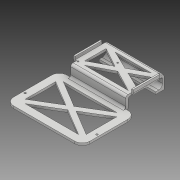
# Autodesk Inventor part: soporte_ubiquiti_usb
Saved by Autodesk Inventor 2018 (Build 220112000, 112)
## iProperties
Created: 2019-01-16
Part Number: soporte_ubiquiti_usb
Material: Genérico
Document SubType Name: Modeling
Designer: becar
Density: 1 g/cm^3
Appearance: Valor por defecto
Author: becar
Autodesk Inventor part; units mm, degrees
ref_plane "YZ Plane" through (0, 0, 0) normal (1, 0, 0) x (0, 1, 0)
ref_plane "XZ Plane" through (0, 0, 0) normal (0, 1, 0) x (-1, 0, 0)
ref_plane "XY Plane" through (0, 0, 0) normal (0, 0, 1) x (1, 0, 0)
sketch "Boceto1" plane through (0, 0, 0) normal (0, 0, 1) x (1, 0, 0)
  line L0 (0, 0) -> (100, 0)
  line L1 (100, 0) -> (100, 70)
  line L2 (100, 70) -> (0, 70)
  line L3 (0, 70) -> (0, 0)
  line L4 (0, 0) -> (0, 22)
  line L5 (100, 0) -> (100, 22)
  circle A0 centre (3, 22) radius 1.25
  circle A1 centre (97, 22) radius 1.25
  line L6 (0, 70) -> (10, 70)
  line L7 (100, 0) -> (90, 0)
  line L8 (90, 0) -> (90, 10)
  line L9 (10, 70) -> (10, 60)
  line L10 (100, 70) -> (90, 70)
  line L11 (90, 70) -> (90, 60)
  line L12 (0, 0) -> (10, 0)
  line L13 (15, 60) -> (85, 60)
  line L14 (15, 10) -> (85, 10)
  line L15 (10, 15) -> (10, 55)
  line L16 (90, 15) -> (90, 55)
  line L17 (10, 55) -> (43.3333, 35)
  line L18 (10, 15) -> (43.3333, 35)
  line L19 (50, 39) -> (15, 60)
  line L20 (50, 39) -> (85, 60)
  line L21 (90, 55) -> (56.6667, 35)
  line L22 (56.6667, 35) -> (90, 15)
  line L23 (85, 10) -> (50, 31)
  line L24 (50, 31) -> (15, 10)
  dimension "d0" = 100
  dimension "d1" = 70
  dimension "d2" = 22
  dimension "d4" = 22
  dimension "d6" = 2.5
  dimension "d7" = 2.5
  dimension "d8" = 10
  dimension "d9" = 10
  dimension "d10" = 10
  dimension "d11" = 10
  dimension "d12" = 5
  dimension "d13" = 5
  dimension "d14" = 5
  dimension "d15" = 5
  dimension "d16" = 10
  constraints: 50 end point, 6 perpendicular, 6 point on line, 2 centre point, 1 collinear, 1 horizontal, 1 vertical
  measures "d0" distance of L0.start L0.end
  measures "d1" distance of L0.end L1.end
  measures "d2" distance of L0.start L4.end
  measures "d4" distance of L0.end L5.end
  measures "d6" diameter of A0
  measures "d7" diameter of A1
  measures "d8" distance of L2.end L6.end
  measures "d9" distance of L0.end L7.end
  measures "d10" distance of L7.end L8.end
  measures "d11" distance of L6.end L9.end
  measures "d12" distance of L9.end L15.end
  measures "d13" distance of L8.end L14.end
  measures "d14" distance of L9.end L13.start
  measures "d15" distance of L8.end L16.start
  measures "d16" distance of L1.end L10.end
extrude "Extrusión1" add sketch "Boceto1" along normal blind 3
sketch "Boceto2" plane through (100, 0, 0) normal (1, 0, 0) x (0, 0, -1)
  line L0 (-3, 70) -> (-3, 0) projected
  line L1 (-3, 70) -> (-18, 70)
  line L2 (-18, 70) -> (-18, 120)
  line L3 (-18, 120) -> (0, 120)
  line L4 (0, 120) -> (0, 117)
  line L5 (0, 117) -> (0, 109)
  line L6 (0, 109) -> (-3, 109)
  line L7 (-3, 109) -> (-3, 117)
  line L8 (-3, 117) -> (-15, 117)
  line L9 (-15, 117) -> (-15, 73)
  line L10 (-15, 73) -> (0, 73)
  line L11 (0, 73) -> (0, 70)
  line L12 (0, 70) -> (-3, 70) projected
  line L13 (0, 70) -> (-3, 70)
  point P0 (0, 0)
  dimension "d25" = 15
  dimension "d26" = 50
  dimension "d27" = 3
  dimension "d28" = 8
  dimension "d29" = 3
  dimension "d30" = 12
  dimension "d31" = 44
  constraints: 24 end point, 6 perpendicular, 3 point on line, 2 vertical, 1 collinear, 1 horizontal
  measures "d25" distance of L0.start L1.end
  measures "d26" distance of L1.end L2.end
  measures "d27" distance of L3.end L4.end
  measures "d28" distance of L4.end L5.end
  measures "d29" distance of L5.end L6.end
  measures "d30" distance of L7.end L8.end
  measures "d31" distance of L8.end L9.end
extrude "Extrusión2" add sketch "Boceto2" against normal up to surface (100 mm away)
sketch "Boceto3" plane through (100, 70, 18) normal (0, 0, 1) x (1, 0, 0)
  line L0 (0, 50) -> (-100, 50) projected
  line L1 (-50, 50) -> (-87, 50)
  line L2 (-87, 50) -> (-87, -0.2579)
  line L3 (-87, -0.2579) -> (-100, -0.2579)
  line L4 (-100, -0.2579) -> (-100, 50)
  line L5 (-100, 50) -> (-87, 50)
  line L6 (-50, 50) -> (-13, 50)
  line L7 (-13, 50) -> (-13, -0.2579)
  line L8 (-13, -0.2579) -> (0, -0.2579)
  line L9 (0, -70) -> (0, 3) projected
  line L10 (0, -0.2579) -> (0, 50)
  line L11 (-13, 50) -> (0, 50)
  point P0 (-100, -70)
  dimension "d34" = 37
  dimension "d35" = 37
  constraints: 20 end point, 7 perpendicular, 3 point on line, 1 horizontal, 1 midpoint
  measures "d34" distance of L1.start L1.end
  measures "d35" distance of L1.start L6.end
extrude "Extrusión3" cut sketch "Boceto3" against normal up to surface (18 mm away)
sketch "Boceto4" plane through (13, 120, 18) normal (0, 0, 1) x (1, 0, 0)
  line L0 (0, 0) -> (0, -50) projected
  line L1 (0, -25) -> (0, -7.5)
  line L2 (0, -7.5) -> (-2, -7.5)
  line L3 (-2, -7.5) -> (-2, -42.5)
  line L4 (-2, -42.5) -> (0, -42.5)
  line L5 (0, -42.5) -> (0, -25)
  line L6 (74, -50) -> (74, 0) projected
  line L7 (74, -25) -> (74, -7.5)
  line L8 (74, -7.5) -> (76, -7.5)
  line L9 (76, -7.5) -> (76, -42.5)
  line L10 (76, -42.5) -> (74, -42.5)
  line L11 (74, -42.5) -> (74, -25)
  point P0 (-13, -120)
  dimension "d38" = 17.5
  dimension "d39" = 2
  dimension "d40" = 35
  dimension "d41" = 2
  constraints: 20 end point, 6 perpendicular, 4 point on line, 2 collinear, 2 midpoint
  measures "d38" distance of L1.start L1.end
  measures "d39" distance of L1.end L2.end
  measures "d40" distance of L2.end L3.end
  measures "d41" distance of L7.end L8.end
extrude "Extrusión4" add sketch "Boceto4" along normal blind 4
sketch "Boceto5" plane through (87, 77.5, 18) normal (0, -1, 0) x (1, 0, 0)
  line L0 (-76, 0) -> (-76, -3)
  line L1 (0, -3) -> (-74, -3) projected
  line L2 (-76, -3) -> (-74, -3)
  line L3 (0, 0) -> (-74, 0) projected
  line L4 (-74, -3) -> (-74, 0)
  line L5 (0, 0) -> (2, 0) projected
  line L6 (2, 0) -> (2, -3)
  line L7 (0, -3) -> (0, -18) projected
  line L8 (2, -3) -> (0, -3)
  line L9 (0, -3) -> (0, 0)
  line L10 (0, 0) -> (2, 0)
  line L11 (-76, 0) -> (-76, 4) projected
  line L12 (-76, 0) -> (-74, 0) projected
  line L13 (-76, 0) -> (-74, 0)
  point P0 (-87, -18)
  dimension "d44" = 3
  constraints: 16 end point, 4 perpendicular, 2 vertical, 1 collinear
  measures "d44" distance of L0.start L0.end
extrude "Extrusión5" add sketch "Boceto5" against normal up to surface (35 mm away) contours L12 L4 L2 L0 | L5 L6 L8 L9
sketch "Boceto6" plane through (13, 120, 18) normal (0, 0, 1) x (1, 0, 0)
  line L0 (74, 0) -> (0, 0) projected
  line L1 (37, 0) -> (1.25, 0)
  line L2 (37, 0) -> (72.75, 0)
  line L3 (72.75, 0) -> (72.75, -47)
  line L4 (74, -47) -> (0, -47) projected
  line L5 (72.75, -23.5) -> (72.75, -2)
  line L6 (72.75, -23.5) -> (72.75, -45)
  line L7 (72.75, -45) -> (1.25, -45)
  line L8 (1.25, -45) -> (1.25, -2)
  line L9 (1.25, -2) -> (72.75, -2)
  line L10 (1.25, -2) -> (1.25, -18)
  line L11 (1.25, -18) -> (31.25, -18)
  circle A0 centre (31.25, -18) radius 1
  line L12 (1.25, -45) -> (3.75, -45)
  line L13 (3.75, -45) -> (3.75, -42.5)
  circle A1 centre (3.75, -42.5) radius 1
  line L14 (72.75, -2) -> (71.25, -2)
  line L15 (71.25, -2) -> (71.25, -3.5)
  circle A2 centre (71.25, -3.5) radius 1
  point P0 (-13, -120)
  dimension "d47" = 35.75
  dimension "d48" = 35.75
  dimension "d49" = 21.5
  dimension "d50" = 21.5
  dimension "d52" = 16
  dimension "d53" = 30
  dimension "d54" = 2
  dimension "d55" = 2.5
  dimension "d56" = 2.5
  dimension "d57" = 2
  dimension "d58" = 1.5
  dimension "d59" = 1.5
  dimension "d60" = 2
  constraints: 28 end point, 8 point on line, 6 perpendicular, 3 centre point, 3 coincident, 2 midpoint
  measures "d47" distance of L1.start L1.end
  measures "d48" distance of L1.start L2.end
  measures "d49" distance of L5.start L5.end
  measures "d50" distance of L5.start L6.end
  measures "d52" distance of L8.end L10.end
  measures "d53" distance of L10.end L11.end
  measures "d54" diameter of A0
  measures "d55" distance of L7.end L12.end
  measures "d56" distance of L12.end L13.end
  measures "d57" diameter of A1
  measures "d58" distance of L5.end L14.end
  measures "d59" distance of L14.end L15.end
  measures "d60" diameter of A2
extrude "Extrusión6" cut sketch "Boceto6" against normal up to surface (3 mm away) contours A0 | A1 | A2
move faces "Desplazar1" translate (0, 1, 0) faces at (61.128, 117, 7)
move faces "Desplazar2" translate (2, 0, 0) faces at (13, 72, 6)
move faces "Desplazar3" translate (0, -0.25, 0) faces at (39, 70, 13)
sketch "Boceto7" plane through (13, 120, 18) normal (0, 0, 1) x (1, 0, 0)
  line L0 (0, -7.5) -> (0, -42.5) projected
  line L1 (0, 0) -> (0, -7.5)
  line L2 (77, -7.5) -> (72, -7.5)
  line L3 (0, -7.5) -> (7.5, -7.5)
  line L4 (77, -7.5) -> (69.5, -7.5)
  line L5 (69.5, -42.5) -> (67.5, -42.5)
  line L6 (7.5, -42.5) -> (7.5, -37.5)
  line L7 (17.5, -7.5) -> (42.0628, -19.309)
  line L8 (42.0628, -19.309) -> (64.5, -7.5)
  line L9 (17.5, -7.5) -> (64.5, -7.5)
  line L10 (49.6407, -22.9523) -> (69.5, -12.5)
  line L11 (69.5, -12.5) -> (69.5, -32.5)
  line L12 (49.6407, -22.9523) -> (69.5, -32.5)
  line L13 (41, -27.5) -> (12.5, -42.5)
  line L14 (12.5, -42.5) -> (67.5, -42.5)
  line L15 (7.5, -37.5) -> (33.5147, -23.8081)
  line L16 (33.5147, -23.8081) -> (7.5, -9.5)
  line L17 (7.5, -9.5) -> (7.5, -37.5)
  line L18 (41, -27.5) -> (69.5, -42.5)
  point P0 (-13, -120)
  dimension "d72" = 5
  dimension "d73" = 7.5
  dimension "d75" = 10
  dimension "d77" = 2
  dimension "d78" = 10
  dimension "d79" = 2
  dimension "d80" = 5
  constraints: 36 end point, 2 collinear, 1 horizontal, 1 parallel
  measures "d72" distance of L2.start L2.end
  measures "d73" distance of L0.start L3.end
  measures "d75" distance of L3.end L7.start
  measures "d77" distance of L3.end L16.end
  measures "d78" distance of L5.start L11.end
  measures "d79" distance of L5.start L5.end
  measures "d80" distance of L6.start L13.end
extrude "Extrusión7" cut sketch "Boceto7" against normal up to surface (3 mm away)
fillet "Empalme1" radius 5 1 edges at (50, 118, 3)
fillet "Empalme2" radius 3 1 edges at (51, 69.75, 3)
fillet "Empalme3" radius 3 4 edges at (51, 69.75, 18) (50, 120, 18) (89, 95, 15) (11, 95, 15)
sketch "Boceto8" plane through (0, 0, 3) normal (0, 0, 1) x (1, 0, 0)
  line L0 (0, 66.75) -> (100, 66.75) projected
  line L1 (0, 66.75) -> (15, 66.75)
  line L2 (15, 69.7421) -> (15, 69.75) projected
  line L3 (15, 66.75) -> (15, 69.75)
  line L4 (15, 69.75) -> (0, 69.7421)
  line L5 (0, 69.7421) -> (0, 66.75)
  line L6 (100, 0) -> (100, 66.75) projected
  line L7 (100, 66.75) -> (86.9947, 66.75)
  line L8 (86.9947, 66.75) -> (86.9947, 69.7421)
  line L9 (100, 0) -> (100, 69.7421) projected
  line L10 (86.9947, 69.7421) -> (100, 69.7421)
  line L11 (100, 69.7421) -> (100, 66.75)
  line L12 (86.9947, 66.75) -> (86.9947, 69.7421)
  point P0 (0, 0)
  dimension "d25" = 15
  dimension "d26" = 50
  dimension "d27" = 3
  dimension "d28" = 8
  dimension "d29" = 3
  dimension "d30" = 12
  dimension "d31" = 44
  constraints: 18 end point, 3 perpendicular, 1 collinear, 1 horizontal, 1 point on line, 1 vertical
extrude "Extrusión8" cut sketch "Boceto8" along normal blind 4
fillet "Empalme4" radius 10 4 edges at (0, 69.7421, 1.5) (0, 0, 1.5) (100, 0, 1.5) (100, 69.7421, 1.5)
fillet "Empalme5" radius 3 1 edges at (51, 73, 0)
fillet "Empalme6" radius 2 3 edges at (13.4927, 118, 15.0432) (86.5073, 118, 15.0432) (50, 118, 15)
fillet "Empalme7" radius 3 2 edges at (86.5073, 73, 15.0432) (50.5, 73, 15)
